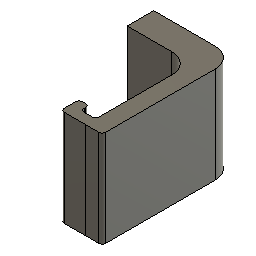
Test_rychka_10% (Autodesk Fusion 360 design; units mm, degrees)
Autodesk Fusion 360 part; units mm, degrees
sketch "Sketch1" plane through (0, 0, 0) normal (0, 1, 0) x (1, 0, 0)
  line L0 (0, 0) -> (203.5, 0)
  line L1 (209.5, -6) -> (209.5, -39)
  line L2 (204.5, -14) -> (204.5, -36)
  line L3 (204.5, -40) -> (208.5, -40)
  line L4 (204.5, -40) -> (198, -40)
  line L5 (203.5, -37) -> (201, -37)
  line L6 (200, -36) -> (200, -35.5)
  line L7 (199, -34.5) -> (198, -34.5)
  line L8 (197, -35.5) -> (197, -39)
  arc A0 (200, -35.5) -> (199, -34.5) centre (199, -35.5) ccw
  arc A1 (198, -34.5) -> (197, -35.5) centre (198, -35.5) ccw
  arc A2 (200, -36) -> (201, -37) centre (201, -36) ccw
  arc A3 (203.5, -37) -> (204.5, -36) centre (203.5, -36) ccw
  arc A4 (197, -39) -> (198, -40) centre (198, -39) ccw
  arc A5 (208.5, -40) -> (209.5, -39) centre (208.5, -39) ccw
  line L9 (0, -8) -> (198.5, -8)
  arc A6 (204.5, -14) -> (198.5, -8) centre (198.5, -14) ccw
  arc A7 (209.5, -6) -> (203.5, 0) centre (203.5, -6) ccw
  line L10 (185, 0) -> (185, -8)
  point P0 (204.5, 0)
  point P1 (209.5, 0)
  point P2 (209.5, -40)
  point P3 (200, -37)
  point P4 (200, -34.5)
  point P5 (197, -34.5)
  point P6 (197, -40)
  dimension "d14" = 5
  dimension "d15" = 40
  dimension "d16" = 7.5
  dimension "d17" = 5.5
  dimension "d18" = 3
  dimension "d20" = 2.5
  dimension "d21" = 1
  dimension "d22" = 1
  dimension "d23" = 1
  dimension "d24" = 1
  dimension "d26" = 6
  dimension "d27" = 6
  constraint coincident L0.start origin
  constraint horizontal L0
  constraint perpendicular L0 L1
  constraint perpendicular L0 L2
  constraint perpendicular L1 L3
  constraint perpendicular L2 L4
  constraint perpendicular L2 L5
  constraint perpendicular L5 L6
  constraint perpendicular L2 L7
  constraint perpendicular L7 L8
  constraint coincident P4 L6
  constraint coincident P4 L7
  constraint tangent L6 A0
  constraint tangent L7 A0
  constraint coincident P5 L7
  constraint coincident P5 L8
  constraint tangent L7 A1
  constraint tangent L8 A1
  constraint equal A0 A1
  constraint coincident P3 L5
  constraint coincident P3 L6
  constraint tangent L5 A2
  constraint tangent L6 A2
  constraint coincident L3.start L2
  constraint tangent L2 A3
  constraint tangent L5 A3
  constraint coincident P6 L8
  constraint coincident L4 P6
  constraint tangent L8 A4
  constraint tangent L4 A4
  constraint coincident P2 L1
  constraint coincident P2 L3
  constraint tangent L1 A5
  constraint tangent L3 A5
  constraint equal A4 A5
  constraint coincident P0 L2
  constraint tangent L9 A6
  constraint tangent L2 A6
  constraint coincident P1 L0
  constraint coincident P1 L1
  constraint tangent L0 A7
  constraint tangent L1 A7
  constraint coincident L0 L10.start
  constraint coincident L9 L10.end
  constraint perpendicular L9 L10
  measures "d14" distance of P0 P1
  measures "d15" distance of P1 P2
  measures "d16" distance of L3.start P6
  measures "d17" distance of P5 P6
  measures "d18" distance of P4 P5
  measures "d20" distance of P3 P4
  measures "d21" radius of A0
  measures "d22" radius of A2
  measures "d23" radius of A3
  measures "d24" radius of A4
  measures "d26" radius of A6
  measures "d27" radius of A7
extrude "Extrude1" add sketch "Sketch1" along normal blind 29
